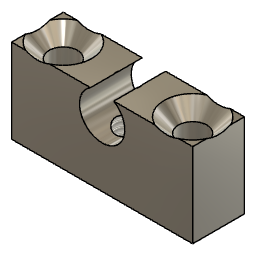
electrode puck v2 connector fixture v10 (Autodesk Fusion 360 design; units mm, degrees)
Autodesk Fusion 360 part; units mm, degrees
sketch "Sketch1" plane through (0, 0, 0) normal (0, 0, 1) x (1, 0, 0)
  circle A0 centre (0, 5) radius 1.75
  line L0 (-7, 6.5) -> (7, 6.5)
  line L1 (7, 6.5) -> (7, 0)
  line L2 (7, 0) -> (-7, 0)
  line L3 (-7, 0) -> (-7, 6.5)
  line L4 (0, 2.5) -> (0, 20) construction
  dimension "d1" = 3.5
  dimension "d2" = 5
  dimension "d3" = 14
  dimension "d4" = 6.5
  constraint vertical origin A0.centre
  constraint horizontal L0
  constraint vertical L1
  constraint horizontal L2
  constraint vertical L3
  constraint symmetric L1 L3 L4
  constraint coincident origin L2
  measures "d1" diameter of A0
  measures "d2" distance of origin A0.centre
  measures "d3" distance of L0.start L0.end
  measures "d4" distance of L0 L2
extrude "Extrude1" add sketch "Sketch1" against normal blind 4 contours A0 L0 L1 L2 L3
sketch "Sketch3" plane through (0, 6.5, 0) normal (0, 1, 0) x (-1, 0, 0)
  line L0 (-0.9014, 0) -> (-7, 0)
  line L1 (-7, 0) -> (-7, -4)
  line L2 (-7, -4) -> (-0.9014, -4)
  line L3 (7, -4) -> (7, 0)
  line L4 (7, -2) -> (-7, -2) construction
  line L5 (0, 0) -> (0, -4.5) construction
  line L6 (-0.9014, -4) -> (-0.9014, 0)
  line L7 (7, 0) -> (0.9014, 0)
  line L8 (0.9014, 0) -> (0.9014, -4)
  line L9 (0.9014, -4) -> (7, -4)
  point P0 (5, -2)
  point P1 (-5, -2)
  dimension "d7" = 10
  constraint midpoint L3 L4.start
  constraint midpoint L1 L4.end
  constraint coincident L4 P0
  constraint coincident L4 P1
  constraint coincident L5.start origin
  constraint symmetric P0 P1 L5
  measures "d7" distance of P0 P1
hole "Hole1" at (5, 6.5, -2) at (-5, 6.5, -2) direction (0, -1, 0) diameter 2.2 end through all countersink diameter 4.4 countersink angle 90
hole "Hole2" at (0, 0, -2) direction (0, 1, 0) diameter 1.875 depth 7.5 tip angle 118
thread "Thread1" "ISO Metric profile 2.3 M2.3x0.45 6H" thread offset 0 thread depth 10
